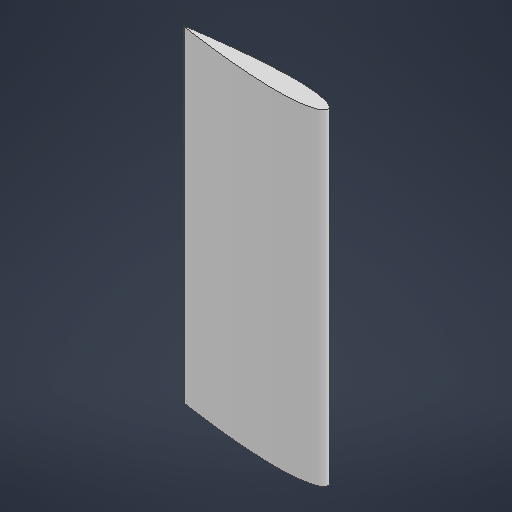
# Autodesk Inventor part: Delb_Tail_v1
Saved by Autodesk Inventor 2026 (Build 300175050, 175E)
## iProperties
Created: 2026-06-09
Part Number: Delb_Tail_v1
Material: Generic
Document SubType Name: Modeling
Designer: Delbe
Density: 1 g/cm^3
Appearance: Default
Author: Delbe
Autodesk Inventor part; units mm, degrees
ref_plane "YZ Plane" through (0, 0, 0) normal (1, 0, 0) x (0, 1, 0)
ref_plane "XZ Plane" through (0, 0, 0) normal (0, 1, 0) x (-1, 0, 0)
ref_plane "XY Plane" through (0, 0, 0) normal (0, 0, 1) x (1, 0, 0)
sketch "Sketch1" plane through (0, 0, 0) normal (0, 1, 0) x (-1, 0, 0)
  spline S0 degree 4 poles (200, 0.283) (199.9285, 0.2943) (199.5798, 0.3492) (198.995, 0.441) (198.0088, 0.595) (196.9736, 0.7557) (195.7049, 0.9513) (194.215, 1.179) (192.5035, 1.4381) (190.5765, 1.7267) (188.4374, 2.0431) (186.0919, 2.3855) (183.5453, 2.7519) (180.8035, 3.1403) (177.8729, 3.5487) (174.7605, 3.9749) (171.4734, 4.4167) (168.0194, 4.8719) (164.4065, 5.3383) (160.6432, 5.8137) (156.7382, 6.2957) (152.7008, 6.7822) (148.5402, 7.2707) (144.2663, 7.7589) (139.889, 8.2445) (135.4185, 8.7248) (130.8653, 9.1974) (126.2401, 9.6598) (121.5535, 10.1091) (116.8166, 10.5428) (112.0404, 10.958) (107.2361, 11.3518) (102.4149, 11.7214) (97.588, 12.0639) (92.7668, 12.3763) (87.9623, 12.6557) (83.1863, 12.8994) (78.4483, 13.1045) (73.763, 13.2685) (69.1296, 13.389) (64.5937, 13.4633) (60.0731, 13.4906) (55.744, 13.4671) (51.4536, 13.3935) (47.2992, 13.2675) (43.2599, 13.0888) (39.3548, 12.8569) (35.5903, 12.5719) (31.9763, 12.2341) (28.521, 11.8445) (25.2324, 11.404) (22.1181, 10.9143) (19.1854, 10.377) (16.441, 9.7944) (13.8911, 9.1686) (11.5415, 8.5021) (9.3973, 7.7972) (7.4632, 7.0568) (5.7427, 6.2829) (4.2399, 5.4776) (2.9546, 4.6424) (1.8949, 3.7771) (1.0489, 2.8811) (0.4553, 1.9508) (0.0446, 0.991) (0.0199, 0.0001) (0.0446, -0.9911) (0.4553, -1.9508) (1.0489, -2.8811) (1.8949, -3.7771) (2.9546, -4.6424) (4.2399, -5.4776) (5.7427, -6.2829) (7.4632, -7.0568) (9.3973, -7.7972) (11.5415, -8.5021) (13.8911, -9.1686) (16.441, -9.7944) (19.1854, -10.377) (22.1181, -10.9143) (25.2324, -11.404) (28.521, -11.8445) (31.9763, -12.2341) (35.5903, -12.5719) (39.3548, -12.8569) (43.2599, -13.0888) (47.2992, -13.2675) (51.4536, -13.3934) (55.744, -13.4672) (60.0731, -13.4903) (64.5937, -13.4635) (69.1296, -13.389) (73.763, -13.2685) (78.4483, -13.1045) (83.1863, -12.8994) (87.9623, -12.6557) (92.7668, -12.3763) (97.588, -12.0639) (102.4149, -11.7214) (107.2361, -11.3518) (112.0404, -10.958) (116.8166, -10.5428) (121.5535, -10.1091) (126.2401, -9.6598) (130.8653, -9.1974) (135.4185, -8.7248) (139.889, -8.2445) (144.2663, -7.7589) (148.5402, -7.2707) (152.7008, -6.7822) (156.7382, -6.2957) (160.6432, -5.8137) (164.4065, -5.3383) (168.0194, -4.8719) (171.4734, -4.4167) (174.7605, -3.9749) (177.8729, -3.5487) (180.8035, -3.1403) (183.5453, -2.7519) (186.0919, -2.3855) (188.4374, -2.0431) (190.5765, -1.7267) (192.5035, -1.4381) (194.215, -1.179) (195.7049, -0.9513) (196.9736, -0.7557) (198.0088, -0.595) (198.995, -0.441) (199.5798, -0.3492) (199.9285, -0.2943) (200, -0.283) knots 0 0 0 0 0 0.006289 0.00999 0.014294 0.019117 0.024398 0.030094 0.036169 0.042594 0.049343 0.056393 0.063723 0.071314 0.079149 0.087211 0.095485 0.103956 0.112609 0.121431 0.130407 0.139526 0.148774 0.158138 0.167607 0.177167 0.186807 0.196516 0.206281 0.216089 0.225931 0.235794 0.245666 0.255536 0.265393 0.275225 0.28502 0.294767 0.304455 0.31408 0.323615 0.333056 0.342391 0.351601 0.360692 0.369642 0.378441 0.387075 0.395534 0.403805 0.411875 0.419731 0.427362 0.434753 0.441891 0.448764 0.455357 0.46166 0.467661 0.473355 0.478742 0.483835 0.488665 0.493288 0.497778 0.502222 0.506712 0.511335 0.516165 0.521258 0.526645 0.532339 0.53834 0.544643 0.551236 0.558109 0.565247 0.572638 0.580269 0.588125 0.596195 0.604466 0.612925 0.621559 0.630358 0.639308 0.648399 0.657609 0.666944 0.676385 0.68592 0.695545 0.705233 0.71498 0.724775 0.734607 0.744464 0.754334 0.764206 0.774069 0.783911 0.793719 0.803484 0.813193 0.822833 0.832393 0.841862 0.851226 0.860474 0.869593 0.878569 0.887391 0.896044 0.904515 0.912789 0.920851 0.928686 0.936277 0.943607 0.950657 0.957406 0.963831 0.969906 0.975602 0.980883 0.985706 0.99001 0.993711 1 1 1 1 1
  line L0 (200, 0.283) -> (200, -0.283)
  line L1 (0.0318, 0.0001) -> (60.0318, 0.0001)
  line L2 (60.0318, 0.0001) -> (60.0318, 13.4801)
  line L3 (60.0318, -13.4799) -> (60.0318, 13.4801)
  point P0 (0, 0)
  point P1 (199.8832, 0.3014)
  point P2 (199.5332, 0.3564)
  point P3 (198.9506, 0.4478)
  point P4 (198.137, 0.5749)
  point P5 (197.0942, 0.7368)
  point P6 (195.8246, 0.9325)
  point P7 (194.3312, 1.1608)
  point P8 (192.6175, 1.4203)
  point P9 (190.6874, 1.7094)
  point P10 (188.5456, 2.0263)
  point P11 (186.197, 2.3692)
  point P12 (183.647, 2.7361)
  point P13 (180.9017, 3.1252)
  point P14 (177.9674, 3.5341)
  point P15 (174.8511, 3.9609)
  point P16 (171.5599, 4.4033)
  point P17 (168.1016, 4.8592)
  point P18 (164.4842, 5.3262)
  point P19 (160.7163, 5.8022)
  point P20 (156.8065, 6.2849)
  point P21 (152.764, 6.772)
  point P22 (148.5983, 7.2612)
  point P23 (144.3192, 7.75)
  point P24 (139.9365, 8.2361)
  point P25 (135.4605, 8.7169)
  point P26 (130.9017, 9.19)
  point P27 (126.2707, 9.6528)
  point P28 (121.5784, 10.1026)
  point P29 (116.8357, 10.5365)
  point P30 (112.0537, 10.9519)
  point P31 (107.2435, 11.3459)
  point P32 (102.4164, 11.7156)
  point P33 (97.5836, 12.058)
  point P34 (92.7565, 12.3703)
  point P35 (87.9463, 12.6495)
  point P36 (83.1643, 12.8928)
  point P37 (78.4216, 13.0974)
  point P38 (73.7293, 13.2608)
  point P39 (69.0983, 13.3805)
  point P40 (64.5395, 13.4542)
  point P41 (55.6808, 13.4558)
  point P42 (51.4017, 13.3807)
  point P43 (47.236, 13.2532)
  point P44 (43.1935, 13.0728)
  point P45 (39.2837, 12.839)
  point P46 (35.5158, 12.5519)
  point P47 (31.8984, 12.2118)
  point P48 (28.4401, 11.8196)
  point P49 (25.1489, 11.3763)
  point P50 (22.0326, 10.8834)
  point P51 (19.0983, 10.3426)
  point P52 (16.353, 9.756)
  point P53 (13.803, 9.1257)
  point P54 (11.4544, 8.4543)
  point P55 (9.3126, 7.744)
  point P56 (7.3825, 6.9976)
  point P57 (5.6688, 6.2175)
  point P58 (4.1754, 5.4063)
  point P59 (2.9058, 4.5661)
  point P60 (1.863, 3.6993)
  point P61 (1.0494, 2.8077)
  point P62 (0.4668, 1.8931)
  point P63 (0.1168, 0.9569)
  point P64 (0.1168, -0.9569)
  point P65 (0.4668, -1.8931)
  point P66 (1.0494, -2.8077)
  point P67 (1.863, -3.6993)
  point P68 (2.9058, -4.5661)
  point P69 (4.1754, -5.4063)
  point P70 (5.6688, -6.2175)
  point P71 (7.3825, -6.9976)
  point P72 (9.3126, -7.744)
  point P73 (11.4544, -8.4543)
  point P74 (13.803, -9.1257)
  point P75 (16.353, -9.756)
  point P76 (19.0983, -10.3426)
  point P77 (22.0326, -10.8834)
  point P78 (25.1489, -11.3763)
  point P79 (28.4401, -11.8196)
  point P80 (31.8984, -12.2118)
  point P81 (35.5158, -12.5519)
  point P82 (39.2837, -12.839)
  point P83 (43.1935, -13.0728)
  point P84 (47.236, -13.2532)
  point P85 (51.4017, -13.3807)
  point P86 (55.6808, -13.4558)
  point P87 (64.5395, -13.4542)
  point P88 (69.0983, -13.3805)
  point P89 (73.7293, -13.2608)
  point P90 (78.4216, -13.0974)
  point P91 (83.1643, -12.8928)
  point P92 (87.9463, -12.6495)
  point P93 (92.7565, -12.3703)
  point P94 (97.5836, -12.058)
  point P95 (102.4164, -11.7156)
  point P96 (107.2435, -11.3459)
  point P97 (112.0537, -10.9519)
  point P98 (116.8357, -10.5365)
  point P99 (121.5784, -10.1026)
  point P100 (126.2707, -9.6528)
  point P101 (130.9017, -9.19)
  point P102 (135.4605, -8.7169)
  point P103 (139.9365, -8.2361)
  point P104 (144.3192, -7.75)
  point P105 (148.5983, -7.2612)
  point P106 (152.764, -6.772)
  point P107 (156.8065, -6.2849)
  point P108 (160.7163, -5.8022)
  point P109 (164.4842, -5.3262)
  point P110 (168.1016, -4.8592)
  point P111 (171.5599, -4.4033)
  point P112 (174.8511, -3.9609)
  point P113 (177.9674, -3.5341)
  point P114 (180.9017, -3.1252)
  point P115 (183.647, -2.7361)
  point P116 (186.197, -2.3692)
  point P117 (188.5456, -2.0263)
  point P118 (190.6874, -1.7094)
  point P119 (192.6175, -1.4203)
  point P120 (194.3312, -1.1608)
  point P121 (195.8246, -0.9325)
  point P122 (197.0942, -0.7368)
  point P123 (198.137, -0.5749)
  point P124 (198.9506, -0.4478)
  point P125 (199.5332, -0.3564)
  point P126 (199.8832, -0.3014)
  dimension "d0" = 60
  dimension "d1" = 26.9599
  constraints: 8 end point, 2 perpendicular, 1 collinear, 1 vertical, 131 other
  measures "d0" distance of L1.start L1.end
  measures "d1" distance of L3.start L2.end
extrude "Extrusion1" add sketch "Sketch1" along normal blind 453.491
body "Solid1"
